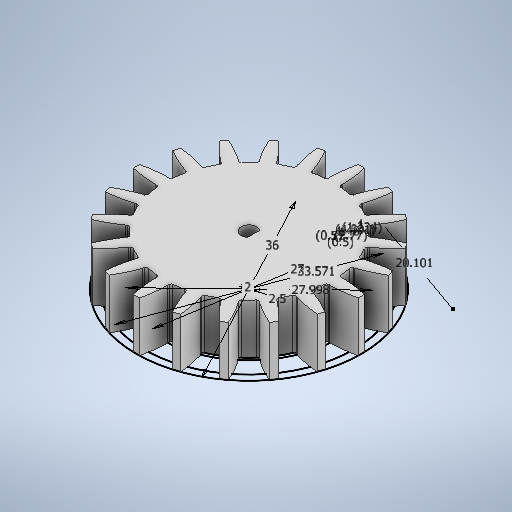
# Autodesk Inventor part: FINmotorgear
Saved by Autodesk Inventor 2025.2 (Build 292293000, 293)
## iProperties
Created: 2025-02-13
Part Number: FINmotorgear
Material: Generic
Document SubType Name: Modeling
Designer: Teamaerosal
Density: 1 g/cm^3
Appearance: Default
Author: Teamaerosal
Autodesk Inventor part; units mm, degrees
ref_plane "YZ Plane" through (0, 0, 0) normal (1, 0, 0) x (0, 1, 0)
ref_plane "XZ Plane" through (0, 0, 0) normal (0, 1, 0) x (-1, 0, 0)
ref_plane "XY Plane" through (0, 0, 0) normal (0, 0, 1) x (1, 0, 0)
sketch "Sketch1" plane through (0, 0, 0) normal (0, 1, 0) x (-1, 0, 0)
  circle A0 centre (0, 0) radius 18
  circle A1 centre (0, 0) radius 16.7855
  circle A2 centre (0, 0) radius 13.999
  line L0 (0, -13.999) -> (0, 0) construction
  line L1 (0, 0) -> (13.999, 0) construction
  circle A3 centre (0, 0) radius 13.5
  arc A4 (0.5001, -17.9931) -> (1, -13.9632) centre (-19.096, -13.5161) ccw
  arc A5 (-1, -13.9632) -> (-0.5001, -17.9931) centre (19.096, -13.5161) ccw
  line L2 (-1, -13.9632) -> (-1, -13.4629)
  line L3 (1, -13.9632) -> (1, -13.4629)
  arc A6 (-0.75, -1) -> (-0.75, 1) centre (0, 0) ccw
  line L4 (-0.75, -1) -> (-0.75, 1)
  point P0 (0, -16.7855)
  point P1 (0, -16.7855)
  point P2 (0.74, -16.7692)
  point P3 (-0.74, -16.7692)
  point P4 (-0.4999, -17.9931)
  point P5 (-3.765, -17.6018)
  point P6 (0.5138, -17.9927)
  point P7 (-0.5138, -17.9927)
  point P8 (0, -18)
  point P9 (-1, -13.9632)
  point P10 (-0.5001, -17.9931)
  point P11 (1.25, 0)
  dimension "d0" = 36
  dimension "d1" = 33.571
  dimension "d2" = 27.998
  dimension "d3" = 1.48
  dimension "d4" = 27
  dimension "d13" = 20.101
  dimension "d14" = 1
  dimension "d16" = 1
  dimension "d17" = 4.001
  dimension "d18" = 1.2239
  dimension "d19" = 2.7702
  dimension "d23" = 0.5003
  dimension "d24" = 0.5003
  dimension "d28" = 2.5
  dimension "d29" = 2
  constraints: 24 point on circle, 10 end point, 7 centre point, 7 coincident, 4 vertical, 3 symmetric about line, 1 horizontal alignment, 1 perpendicular, 1 vertical alignment, 1 other
  measures "d0" diameter of A0
  measures "d1" diameter of A1
  measures "d2" diameter of A2
  measures "d3" distance of point (0.74, -16.769) point (-0.74, -16.769)
  measures "d4" diameter of A3
  measures "d13" radius of A4
  measures "d14" distance from line of L3.start L0
  measures "d16" distance of A0.end A0.start
  measures "d17" distance of point (0, -18) point (0, -13.999)
  measures "d18" vertical distance of point (-0.74, -16.769) A0.start
  measures "d19" vertical distance of point (-0.74, -16.769) L0.start
  measures "d23" distance of L3.end L3.start
  measures "d24" distance of L2.end point (-1, -13.963)
  measures "d28" diameter of A6
  measures "d29" distance from line of point (1.25, 0) L4
extrude "Extrusion1" add sketch "Sketch1" along normal blind 8 contours A5 A1 A4 A0 | A5 A2 A4 A1 | L2 A3 L3 A2 | A3 | L4 A6 picked at (-0.0822, -17.3191) picked at (-0.2901, -15.2142) picked at (0.7779, -13.6407)
fillet "Fillet1" radius 0.3 2 edges at (1, 4, -13.4629) (-1, 4, -13.4629)
pattern_circular "Circular Pattern1" count 20 over 360 about axis through (0, 0, 0) along (0, 1, 0) of "Extrusion1", "Fillet1"
extrude "Extrusion2" cut sketch "Sketch1" along normal through all contours L4 A6
extrude "Extrusion4" cut sketch "Sketch1" against normal blind 10 contours L4 A6
body "Solid1"
